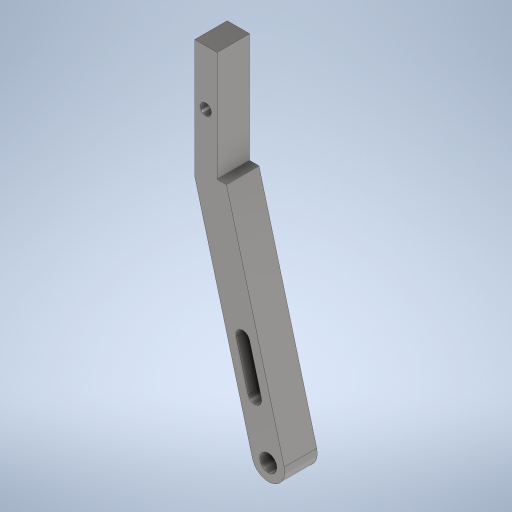
# Autodesk Inventor part: Część ramienia chwytaka
Saved by Autodesk Inventor 2024.1 (Build 281209000, 209)
## iProperties
Created: 2024-05-12
Part Number: Część ramienia chwytaka
Material: Stal, węglowa
Document SubType Name: Modeling
Designer: Krzysiu
Density: 7.85 g/cm^3
Appearance: Częściowo polerowany
Stock Number: 03
Mass: 66.5978 g
Surface Area: 46.7411 cm^2
Volume: 8.48379 cm^3
Author: Krzysiu
Autodesk Inventor part; units mm, degrees
ref_plane "YZ Plane" through (0, 0, 0) normal (1, 0, 0) x (0, 1, 0)
ref_plane "XZ Plane" through (0, 0, 0) normal (0, 1, 0) x (-1, 0, 0)
ref_plane "XY Plane" through (0, 0, 0) normal (0, 0, 1) x (1, 0, 0)
sketch "Szkic1" plane through (0, 0, 0) normal (0, 0, 1) x (1, 0, 0)
  line L0 (-34.8351, 36.7052) -> (-34.8351, 54.7052)
  line L1 (-34.8351, 54.7052) -> (0, 54.7052)
  line L2 (-34.8351, 54.7052) -> (-24.8351, 72.0257)
  line L3 (-34.8351, 54.7052) -> (-14.8351, 54.7052) construction
  line L4 (-34.8351, 54.7052) -> (-24.8351, 37.3847)
  line L5 (-34.8351, 54.7052) -> (-14.8351, 54.7052) construction
  circle A0 centre (-25, 0) radius 2.5
  line L6 (0, 0) -> (0, -12)
  line L7 (-18.3168, -26.6133) -> (-17.2354, -28.9778)
  line L8 (-29.7354, -1.6457) -> (-45.5171, 32.862)
  line L9 (-45.5171, 32.862) -> (-48.5127, 50.611)
  line L10 (-45.5171, 32.862) -> (-27.5171, 32.862) construction
  line L11 (-48.5127, 50.611) -> (-28.5127, 50.611) construction
  line L12 (-48.5127, 50.611) -> (-41.5347, 69.3542)
  line L13 (-48.5127, 50.611) -> (-28.5127, 50.611) construction
  line L14 (-17.2354, -28.9778) -> (2.5, -28.9778)
  circle A1 centre (-17.2354, -28.9778) radius 2.5
  line L15 (-19.7354, -28.9778) -> (-24.7354, -28.9778)
  line L16 (19.7354, -28.9778) -> (24.7354, -28.9778)
  circle A2 centre (17.2354, -28.9778) radius 2.5
  line L17 (25, -12) -> (17.2354, -28.9778)
  line L18 (17.2354, -28.9778) -> (2.5, -28.9778)
  line L19 (0, -12) -> (25, -12)
  line L20 (34.8351, 54.7052) -> (24.8351, 37.3847)
  line L21 (34.8351, 36.7052) -> (34.8351, 54.7052)
  line L22 (48.5127, 50.611) -> (35.7696, 35.1962)
  line L23 (45.5171, 32.862) -> (48.5127, 50.611)
  line L24 (45.5171, 32.862) -> (27.5171, 32.862) construction
  circle A3 centre (25, 0) radius 2.5
  line L25 (25, 0) -> (34.8351, 36.7052)
  circle A4 centre (25, -12) radius 2.5
  line L26 (25, -12) -> (45.5171, 32.862)
  line L27 (0, 0) -> (25, 0)
  line L28 (25, 0) -> (17.2354, -28.9778)
  line L29 (25, 0) -> (-5, 0) construction
  line L30 (25, 0) -> (-13, 0) construction
  line L31 (48.5127, 50.611) -> (28.5127, 50.611) construction
  line L32 (48.5127, 50.611) -> (28.5127, 50.611) construction
  line L33 (34.8351, 54.7052) -> (14.8351, 54.7052) construction
  line L34 (34.8351, 54.7052) -> (14.8351, 54.7052) construction
  line L35 (34.8351, 54.7052) -> (0, 54.7052)
  line L36 (48.5127, 50.611) -> (41.5347, 69.3542)
  line L37 (34.8351, 54.7052) -> (24.8351, 72.0257)
  line L38 (-17.2354, -31.4778) -> (-17.2354, -36.4778)
  line L39 (-17.2354, -36.4778) -> (2.5, -36.4778)
  line L40 (-17.2354, -36.4778) -> (-19.7354, -36.4778)
  line L41 (-24.7354, -28.9778) -> (-24.7354, -31.4778)
  line L42 (-17.2354, -26.4778) -> (-17.2354, -26.3778)
  line L43 (-19.245, -21.4778) -> (-19.7354, -21.4778)
  line L44 (-24.7354, -26.4778) -> (-24.7354, -28.9778)
  line L45 (-14.0687, -21.4778) -> (2.5, -21.4778)
  line L46 (17.2354, -21.4778) -> (19.7354, -21.4778)
  line L47 (25, 0) -> (17.2354, -28.9778)
  line L48 (25, -12) -> (17.2354, -28.9778)
  line L49 (24.7354, -26.4778) -> (24.7354, -28.9778)
  line L50 (17.2354, -26.4778) -> (17.2354, -21.4778)
  line L51 (19.7354, -28.9778) -> (24.7354, -28.9778)
  circle A5 centre (17.2354, -28.9778) radius 2.5
  line L52 (24.7354, -28.9778) -> (24.7354, -31.4778)
  line L53 (17.2354, -36.4778) -> (19.7354, -36.4778)
  line L54 (17.2354, -31.4778) -> (17.2354, -36.4778)
  line L55 (17.2354, -28.9778) -> (-2.5, -28.9778)
  line L56 (17.2354, -36.4778) -> (-2.5, -36.4778)
  line L57 (17.2354, -21.4778) -> (-2.5, -21.4778)
  line L58 (-17.2354, -28.9778) -> (-2.5, -28.9778)
  arc A6 (-23.8449, -23.6295) -> (-24.7354, -26.4778) centre (-19.7354, -26.4778) ccw
  arc A7 (-24.7354, -31.4778) -> (-19.7354, -36.4778) centre (-19.7354, -31.4778) ccw
  arc A8 (24.7354, -26.4778) -> (19.7354, -21.4778) centre (19.7354, -26.4778) ccw
  arc A9 (19.7354, -36.4778) -> (24.7354, -31.4778) centre (19.7354, -31.4778) ccw
  circle A10 centre (-17.2354, -28.9778) radius 2.6
  line L59 (-16.5625, -31.4892) -> (-15.9413, -33.8074)
  line L60 (-17.2354, -28.9778) -> (-9.7354, -28.9778) construction
  line L61 (-9.991, -27.0366) -> (58.009, -27.0366) construction
  arc A11 (-22.0651, -30.2719) -> (-12.4058, -27.6837) centre (-17.2354, -28.9778) ccw
  line L62 (-17.2354, -28.9778) -> (-14.724, -28.3048)
  line L63 (-17.2354, -28.9778) -> (-12.2354, -28.9778) construction
  line L64 (-12.4058, -27.6837) -> (-30.0055, 37.9993)
  line L65 (-12.4058, -27.6837) -> (55.5942, -27.6837) construction
  line L66 (-17.2354, -28.9778) -> (-19.7468, -29.6507)
  line L67 (-17.2354, -28.9778) -> (-12.2354, -28.9778) construction
  line L68 (-22.0651, -30.2719) -> (-39.6648, 35.4111)
  line L69 (-36.6214, 36.2266) -> (-34.8351, 36.7052)
  line L70 (-39.6648, 35.4111) -> (-39.6648, 54.7052)
  circle A12 centre (-21.6297, -12.5783) radius 2.6
  line L71 (-21.6297, -12.5783) -> (-19.1183, -11.9054)
  line L72 (-21.6297, -12.5783) -> (-19.0297, -12.5783) construction
  circle A13 centre (-25, 0) radius 2.6
  line L73 (-25, 0) -> (-22.4886, 0.6729)
  line L74 (-19.1183, -11.9054) -> (-22.4886, 0.6729)
  line L75 (-19.1183, -11.9054) -> (-24.1411, -13.2512)
  line L76 (-22.4886, 0.6729) -> (-27.5114, -0.6729)
  line L77 (-27.5114, -0.6729) -> (-24.1411, -13.2512)
  line L78 (-19.1183, -11.9054) -> (-22.4886, 0.6729)
  line L79 (-30.0055, 37.9993) -> (-34.8351, 37.9993)
  line L80 (-34.8351, 54.7052) -> (-34.8351, 64.7052)
  line L81 (-39.6648, 54.7052) -> (-39.6648, 64.7052)
  line L82 (-39.6648, 64.7052) -> (-39.646, 64.7052)
  line L83 (-34.8351, 37.9993) -> (-39.6648, 37.9993)
  line L84 (-39.6648, 37.9993) -> (-39.6648, 71.4113)
  line L85 (-39.6648, 71.4113) -> (-34.8351, 71.4113)
  line L86 (-34.8351, 71.4113) -> (-34.8351, 64.7052)
  line L87 (-48.5127, 50.611) -> (-38.0868, 37.9993)
  line L88 (-36.6214, 36.2266) -> (-35.7696, 35.1962)
  line L89 (-25, 0) -> (-20.9567, -15.0897)
  line L90 (-17.9084, -26.4664) -> (-17.2354, -28.9778)
  line L91 (-17.2354, -28.9778) -> (-17.9084, -26.4664)
  line L92 (-20.9567, -15.0897) -> (-21.6297, -12.5783)
  line L93 (-25, 0) -> (-20.9567, -15.0897)
  line L94 (-17.9084, -26.4664) -> (-16.5625, -31.4892)
  line L95 (0, -12) -> (-16.6082, -12)
  line L96 (-19.0948, -12) -> (-25, -12)
  line L97 (0, 0) -> (-19.8236, 0)
  line L98 (-22.3083, 0) -> (-25, 0)
  line L99 (-25, 0) -> (-22.3083, 0) construction
  line L100 (-19.8236, 0) -> (13, 0) construction
  line L101 (-25, 0) -> (-22.3083, 0) construction
  line L102 (-19.8236, 0) -> (5, 0) construction
  line L103 (-25, 0) -> (-25.6729, 2.5114)
  line L104 (-33.8053, 32.862) -> (-34.8351, 36.7052)
  line L105 (0, 54.7052) -> (-34.8351, 54.7052)
  line L106 (-39.6648, 54.7052) -> (-43.5601, 54.7052)
  point P0 (0, 0)
  point P1 (0, 0)
  point P2 (2.5, 0)
  point P3 (-24.7354, -36.4778)
  point P4 (-17.2354, -21.4778)
  point P5 (-24.7354, -21.4778)
  point P6 (24.7354, -21.4778)
  point P7 (24.7354, -36.4778)
  dimension "d0" = 25
  dimension "d1" = 30
  dimension "d3" = 38
  dimension "d5" = 18
  dimension "d6" = 20
  dimension "d7" = 60
  dimension "d8" = 20
  dimension "d9" = 60
  dimension "d10" = 5
  dimension "d11" = 12
  dimension "d12" = 25
  dimension "d13" = 49.331
  dimension "d14" = 18
  dimension "d15" = 99.58
  dimension "d16" = 20
  dimension "d18" = 20
  dimension "d19" = 69.58
  dimension "d21" = 5
  dimension "d22" = 5
  dimension "d23" = 5
  dimension "d24" = 5
  dimension "d25" = 5
  dimension "d26" = 5
  dimension "d27" = 5
  dimension "d28" = 5
  dimension "d29" = 16.9778
  dimension "d30" = 32.6
  dimension "d31" = 2.4
  dimension "d34" = 15
  dimension "d35" = 105
  dimension "d36" = 165
  dimension "d38" = 16.978
  dimension "d39" = 5.2
  dimension "d40" = 15
  dimension "d41" = 5.2
  dimension "d42" = 10
  dimension "d43" = 33.412
  constraints: 214 end point, 36 symmetric about line, 30 point on line, 26 point on circle, 21 horizontal, 17 perpendicular, 13 coincident, 12 centre point, 11 tangent, 6 equal length, 3 vertical, 1 collinear, 1 horizontal alignment, 1 midpoint, 14 other
  measures "d0" distance of L6.start L89.start
  measures "d1" distance of L89.start L90.end
  measures "d3" distance of L0.start L89.start
  measures "d5" distance of L0.start L0.end
  measures "d6" distance of L0.end L2.end
  measures "d7" angle of L3 L2
  measures "d8" distance of L0.end L4.end
  measures "d9" angle of L4 L5
  measures "d10" diameter of A0
  measures "d11" distance of L6.start L6.end
  measures "d12" distance of L6.end L96.end
  measures "d13" distance of L96.end L8.end
  measures "d14" distance of L8.end L9.end
  measures "d15" angle of L10 L9
  measures "d16" distance of L9.end L88.end
  measures "d18" distance of L9.end L12.end
  measures "d19" angle of L13 L12
  measures "d21" diameter of A1
  measures "d22" distance of L15.start L15.end
  measures "d23" distance of L38.start L38.end
  measures "d24" distance of L42.start point (-17.235, -21.478)
  measures "d25" radius of A6
  measures "d26" radius of A7
  measures "d27" radius of A8
  measures "d28" radius of A9
  measures "d29" vertical distance of L96.end L7.end
  measures "d30" distance of L93.start L94.end
  measures "d31" distance of L59.start L59.end
  measures "d34" angle of L63 L62
  measures "d35" angle of L65 L64
  measures "d36" angle of L66 L67
  measures "d38" distance of L62.start L92.end
  measures "d39" diameter of A12
  measures "d40" angle of L72 L71
  measures "d41" diameter of A13
  measures "d42" distance of L0.end L80.end
  measures "d43" distance of L83.end L84.end
extrude "Wyciągnięcie proste1" add sketch "Szkic1" along normal blind 9.9 contours L79 L64 A11 L14 A10 L15 L68 L70 L83 | A11 L59 A10 L14 | L15 A10 L38 A11 L68 | A11 L38 A10 L59
extrude "Wyciągnięcie proste2" add sketch "Szkic1" along normal blind 9.9 and the other way blind 4.95 contours L83 L87 L70 L81 L84 L85 L86 L80 L0 | L83 L70 L87
sketch "Szkic3" plane through (0, 0, -4.95) normal (0, 0, -1) x (-1, 0, 0)
  line L0 (39.6648, 71.4113) -> (39.6648, 35.4111) projected
  line L1 (30.0055, 37.9993) -> (34.8351, 37.9993) projected
  line L2 (39.6648, 71.4113) -> (34.8351, 71.4113)
  line L3 (34.8351, 71.4113) -> (34.8351, 37.9993)
  line L4 (34.8351, 37.9993) -> (39.6648, 37.9993)
  line L5 (39.6648, 37.9993) -> (39.6648, 71.4113)
  point P0 (0, 0)
  constraints: 8 end point, 2 parallel, 1 horizontal, 1 perpendicular
extrude "Wyciągnięcie proste3" cut sketch "Szkic3" against normal blind 4.95
sketch "Szkic5" plane through (-34.8351, 37.9993, 0) normal (1, 0, 0) x (0, 0, -1)
  line L0 (0, 0) -> (0, 33.412) projected
  line L1 (-9.9, 33.412) -> (0, 33.412)
  line L2 (0, 33.412) -> (0, 0)
  line L3 (0, 0) -> (-9.9, 0)
  line L4 (-9.9, 0) -> (-9.9, 33.412)
  point P0 (0, -37.9993)
  constraints: 8 end point, 2 parallel, 1 horizontal, 1 perpendicular
extrude "Wyciągnięcie proste4" add sketch "Szkic5" along normal blind 2
sketch "Szkic6" plane through (0, 0, 9.9) normal (0, 0, 1) x (1, 0, 0)
  circle A0 centre (-17.2354, -28.9778) radius 2.6 projected
  circle A1 centre (-17.2354, -28.9778) radius 2.6
  circle A2 centre (-22.0673, -10.9449) radius 2.6
  line L0 (-22.4886, 0.6729) -> (-19.1183, -11.9054) projected
  arc A3 (-24.1411, -13.2512) -> (-19.1183, -11.9054) centre (-21.6297, -12.5783) ccw projected
  arc A4 (-24.1411, -13.2512) -> (-19.1183, -11.9054) centre (-21.6297, -12.5783) ccw
  line L1 (-19.1183, -11.9054) -> (-19.5559, -10.272)
  line L2 (-24.1411, -13.2512) -> (-24.5787, -11.6178)
  line L3 (-17.2354, -28.9778) -> (-20.9567, -15.0897)
  line L4 (-21.3944, -13.4563) -> (-22.0673, -10.9449)
  point P0 (0, 0)
  dimension "d56" = 18.669
  constraints: 8 end point, 7 point on circle, 3 centre point, 3 coincident, 3 point on line, 3 tangent, 1 parallel
  measures "d56" distance of L3.start L4.end
extrude "Wyciągnięcie proste5" add sketch "Szkic6" against normal blind 9.9 contours A3 L2 A2 L0
sketch "Szkic7" plane through (0, 0, 9.9) normal (0, 0, 1) x (1, 0, 0)
  point P0 (-36.2498, 54.7053)
hole "Otwór1" at (-36.2498, 54.7053, 9.9) direction (0, 0, -1) diameter 3.4 end through all
sketch "Szkic8" plane through (0, 0, 9.9) normal (0, 0, 1) x (1, 0, 0)
  circle A0 centre (-17.2354, -28.9778) radius 2.6 projected
  circle A1 centre (-17.2354, -28.9778) radius 2.6
  line L0 (-17.2354, -28.9778) -> (-21.3739, -13.5326)
  line L1 (-17.2354, -28.9778) -> (-1.2454, -28.9778) construction
  arc A2 (-23.8854, -14.2056) -> (-18.8625, -12.8597) centre (-21.3739, -13.5326) ccw
  line L2 (-24.5787, -11.6178) -> (-27.5114, -0.6729) projected
  line L3 (-24.5787, -11.6178) -> (-23.8854, -14.2056)
  line L4 (-22.4886, 0.6729) -> (-19.5559, -10.272) projected
  line L5 (-19.5559, -10.272) -> (-18.8625, -12.8597)
  line L6 (-24.5787, -11.6178) -> (-19.5559, -10.272)
  point P0 (0, 0)
  dimension "d66" = 15.99
  dimension "d67" = 105
  dimension "d68" = 5.2
  constraints: 11 end point, 2 centre point, 2 coincident, 2 point on circle, 2 tangent, 1 equal length, 1 horizontal
  measures "d66" distance of L0.start L0.end
  measures "d67" angle of L1 L0
  measures "d68" diameter of A2
extrude "Wyciągnięcie proste6" cut sketch "Szkic8" against normal blind 9.9 contours A2 L3 L6 L5
sketch "Szkic9" plane through (0, 0, 9.9) normal (0, 0, 1) x (1, 0, 0)
  arc A0 (-23.8854, -14.2056) -> (-18.8625, -12.8597) centre (-21.3739, -13.5326) ccw projected
  circle A1 centre (-21.3739, -13.5326) radius 2.1
  arc A2 (-22.4886, 0.6729) -> (-27.5114, -0.6729) centre (-25, 0) ccw projected
  circle A3 centre (-25, 0) radius 2.1
  line L0 (-25, 0) -> (-22.9716, 0.5435)
  line L1 (-25, 0) -> (-22.9, 0) construction
  line L2 (-22.9716, 0.5435) -> (-19.3455, -12.9891)
  line L3 (-23.4024, -14.0761) -> (-27.0284, -0.5435)
  arc A4 (-23.0056, -15.5569) -> (-18.8625, -12.8597) centre (-21.3739, -13.5326) ccw
  line L4 (-18.8625, -12.8597) -> (-22.4886, 0.6729)
  line L5 (-27.5114, -0.6729) -> (-23.8854, -14.2056)
  point P0 (0, 0)
  dimension "d71" = 4.2
  dimension "d72" = 4.2
  dimension "d73" = 15
  constraints: 12 end point, 6 point on circle, 3 centre point, 3 coincident, 3 tangent, 2 point on line, 1 concentric, 1 equal length, 1 horizontal
  measures "d71" diameter of A1
  measures "d72" diameter of A3
  measures "d73" angle of L1 L0
extrude "Wyciągnięcie proste7" add sketch "Szkic9" against normal blind 9.9
